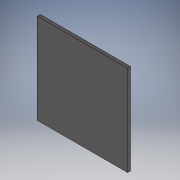
# Autodesk Inventor part: bottom-plate
Saved by Autodesk Inventor 2018 (Build 220112000, 112)
## iProperties
Created: 2024-05-02
Part Number: bottom-plate
Material: Concrete
Document SubType Name: Modeling
Designer: neo
Density: 2.40731 g/cm^3
Appearance: Exposed Aggregate - Coarse
Author: neo
Autodesk Inventor part; units mm, degrees
ref_plane "YZ Plane" through (0, 0, 0) normal (1, 0, 0) x (0, 1, 0)
ref_plane "XZ Plane" through (0, 0, 0) normal (0, 1, 0) x (-1, 0, 0)
ref_plane "XY Plane" through (0, 0, 0) normal (0, 0, 1) x (1, 0, 0)
sketch "Sketch1" plane through (0, 0, 0) normal (0, 1, 0) x (-1, 0, 0)
  line L0 (150, 150) -> (-150, 150)
  line L1 (-150, 150) -> (-150, -150)
  line L2 (-150, -150) -> (150, -150)
  line L3 (150, -150) -> (150, 150)
  circle A0 centre (0, 0) radius 50
  circle A1 centre (20, 0) radius 1.5
  circle A2 centre (0, 0) radius 60
  dimension "d0" = 100
  dimension "d1" = 300
  dimension "d2" = 300
  dimension "d3" = 150
  dimension "d4" = 150
  dimension "d5" = 3
  dimension "d6" = 20
  dimension "d11" = 120
  constraints: 8 end point, 3 centre point, 2 coincident, 2 parallel, 1 horizontal, 1 perpendicular
  measures "d0" diameter of A0
  measures "d1" distance of L2.end L0.start
  measures "d2" distance of L1.end L2.end
  measures "d3" distance from line of L3 point (0, 0)
  measures "d4" distance from line of L0 point (0, 0)
  measures "d5" diameter of A1
  measures "d6" distance of point (0, 0) A1.centre
  measures "d11" diameter of A2
extrude "Extrusion1" add sketch "Sketch1" along normal blind 10 contours L3 L2 L1 L0 | A0 | A1 | A2
extrude "Extrusion2" add sketch "Sketch1" along normal blind 50 contours A1
extrude "Extrusion3" add sketch "Sketch1" along normal blind 18 contours A2
body "Solid1"
